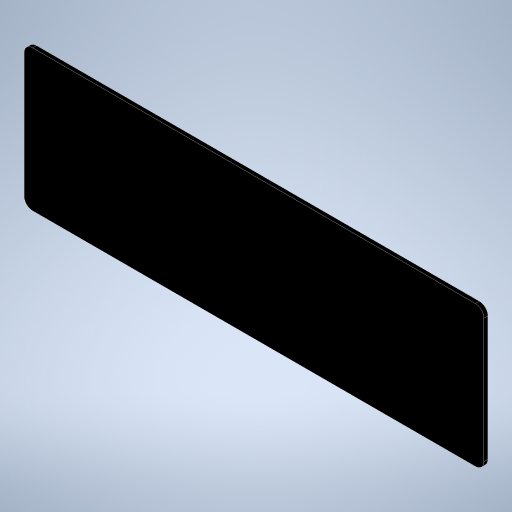
# Autodesk Inventor part: osmobuddy_v1_BOARD
Saved by Autodesk Inventor 2024.3 (Build 283343000, 343)
## iProperties
Created: 2024-08-24
Part Number: osmobuddy_v1_BOARD
Material: Generic
Document SubType Name: Modeling
Designer: atrus
Density: 1 g/cm^3
Appearance: BoardColor
Author: atrus
Autodesk Inventor part; units mm, degrees
ref_plane "YZ Plane" through (0, 0, 0) normal (1, 0, 0) x (0, 1, 0)
ref_plane "XZ Plane" through (0, 0, 0) normal (0, 1, 0) x (-1, 0, 0)
ref_plane "XY Plane" through (0, 0, 0) normal (0, 0, 1) x (1, 0, 0)
ref_plane "BoardFrontPlane" through (0, 0, 0) normal (0, 0, 1) x (1, 0, 0)
sketch "Sketch1" plane through (0, 0, 0) normal (0, 0, 1) x (1, 0, 0)
  line L0 (27, 28) -> (27, 72)
  arc A0 (30, 75) -> (27, 72) centre (30, 72) ccw
  line L1 (30, 75) -> (187, 75)
  arc A1 (190, 72) -> (187, 75) centre (187, 72) ccw
  line L2 (190, 72) -> (190, 28)
  arc A2 (187, 25) -> (190, 28) centre (187, 28) ccw
  line L3 (187, 25) -> (30, 25)
  arc A3 (27, 28) -> (30, 25) centre (30, 28) ccw
  constraints: 8 end point, 8 point on circle, 4 centre point
extrude "BoardOutline" add sketch "Sketch1" along normal blind 1.4202
body "Solid1"
